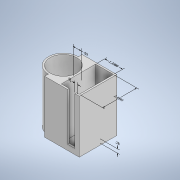
# Autodesk Inventor part: piCaseHolderForMeade
Saved by Autodesk Inventor 2021.2 (Build 252289000, 289)
## iProperties
Created: 2021-02-07
Part Number: piCaseHolderForMeade
Material: Generic
Document SubType Name: Modeling
Designer: robst
Density: 1 g/cm^3
Appearance: Default
Author: robst
Autodesk Inventor part; units mm, degrees
ref_plane "XZ Plane" through (0, 0, 0) normal (0, 1, 0) x (-1, 0, 0)
ref_plane "XY Plane" through (0, 0, 0) normal (0, 0, 1) x (1, 0, 0)
sketch "Sketch1" plane through (0, 0, 0) normal (0, 1, 0) x (-1, 0, 0)
  circle A0 centre (0, 0) radius 25.4
  circle A1 centre (0, 0) radius 28.575
  dimension "d0" = 50.8
  dimension "d1" = 3.175
  constraints: 2 centre point, 2 coincident
  measures "d0" diameter of A0
  measures "d1" radial gap between concentric circles of A0 A1
extrude "Extrusion1" add sketch "Sketch1" against normal blind 100.35
ref_plane "Work Plane1" through (28.575, 0, 0) normal (1, 0, 0) x (0, 1, 0)
sketch "Sketch5" plane through (28.575, 0, 0) normal (1, 0, 0) x (0, 1, 0)
  line L0 (0, 0) -> (-100.35, 0) construction
  line L1 (-100.35, 28.575) -> (-100.35, -28.575) construction
  line L2 (0, -28.575) -> (0, 28.575) projected
  line L3 (-3.175, 0) -> (-3.175, -32.5)
  line L4 (-3.175, -32.5) -> (-97.175, -32.5)
  line L5 (-97.175, -32.5) -> (-97.175, 0)
  line L6 (-3.175, 0) -> (-3.175, 32.5)
  line L7 (-3.175, 32.5) -> (-97.175, 32.5)
  line L8 (-97.175, 32.5) -> (-97.175, 0)
  line L9 (-97.175, 32.5) -> (-3.175, -32.5) construction
  line L10 (-97.175, -32.5) -> (-3.175, 32.5) construction
  line L11 (-100.35, 35.675) -> (-100.35, -35.675)
  line L12 (-100.35, -35.675) -> (0, -35.675)
  line L13 (0, -35.675) -> (0, 35.675)
  line L14 (0, 35.675) -> (-100.35, 35.675)
  line L15 (-100.35, 35.675) -> (0, -35.675) construction
  line L16 (-100.35, -35.675) -> (0, 35.675) construction
  point P0 (-50.175, 0)
  dimension "d7" = 3.175
  dimension "d8" = 32.5
  dimension "d9" = 94
  dimension "d10" = 3.175
  dimension "d11" = 3.175
  constraints: 30 end point, 4 midpoint, 3 parallel, 3 perpendicular, 2 symmetric about line, 2 vertical, 1 point on line
  measures "d7" distance between parallel lines of L3 L2
  measures "d8" distance from line of L3.end L0
  measures "d9" distance of L3.end L4.end
  measures "d10" distance between parallel lines of L13 L6
  measures "d11" distance between parallel lines of L14 L7
extrude "Extrusion2" add sketch "Sketch5" along normal blind 34
sketch "Sketch6" plane through (0, 0, 0) normal (0, 1, 0) x (-1, 0, 0)
  circle A0 centre (0, 0) radius 28.575 projected
  line L0 (-28.575, -35.675) -> (-28.575, 0) projected
  circle A1 centre (0, 0) radius 28.575 projected
  line L1 (-28.575, 0) -> (-28.575, 48.654)
  line L2 (-28.575, 35.675) -> (-62.575, 35.675) projected
  line L3 (-28.575, 48.654) -> (-28.575, 35.675)
  line L4 (-28.575, 35.675) -> (-28.575, 0)
  line L5 (-28.575, 0) -> (-28.575, -35.675)
  line L6 (-28.575, -35.675) -> (-62.575, -35.675) projected
  line L7 (-28.575, -35.675) -> (-28.575, 35.675)
  line L8 (-28.575, 35.675) -> (0, 28.575)
  line L9 (-28.575, 35.675) -> (-28.575, -35.675) projected
  line L10 (-28.575, -35.675) -> (0, -28.575)
  arc A2 (0, 28.575) -> (0, -28.575) centre (0, 0) ccw
  point P0 (0, 28.575)
  point P1 (-28.575, 0)
  point P2 (0, -28.575)
  constraints: 14 end point, 5 point on circle, 3 collinear, 3 vertical, 1 centre point, 1 coincident, 1 concentric, 1 other
extrude "Extrusion3" add sketch "Sketch6" against normal blind 100.35 contours A0 L1 L8 | L10 L0 A0
sketch "Sketch8" plane through (62.575, 0, 0) normal (1, 0, 0) x (0, 0, -1)
  line L0 (-35.675, 0) -> (-35.675, -100.35) projected
  line L1 (35.675, -100.35) -> (35.675, 0) projected
  line L2 (-35.675, -100.35) -> (35.675, -100.35)
  line L3 (35.675, -100.35) -> (35.675, 0)
  line L4 (35.675, 0) -> (-35.675, 0)
  line L5 (-35.675, 0) -> (-35.675, -100.35)
  point P0 (0, 0)
  point P1 (35.675, -100.35)
  point P2 (-35.675, 0)
  constraints: 8 end point, 2 parallel, 1 horizontal, 1 perpendicular
extrude "Extrusion4" add sketch "Sketch8" along normal blind 3.175
sketch "Sketch9" plane through (0, 0, 0) normal (0, 1, 0) x (1, 0, 0)
  line L0 (62.575, -32.5) -> (62.575, 32.5) projected
  line L1 (28.575, 32.5) -> (62.575, 32.5) projected
  line L2 (28.575, -32.5) -> (28.575, 32.5) projected
  line L3 (28.575, -32.5) -> (62.575, -32.5) projected
  line L4 (28.575, 32.5) -> (28.575, -32.5) projected
  line L5 (28.575, -32.5) -> (62.575, -32.5)
  line L6 (62.575, -32.5) -> (62.575, 32.5)
  line L7 (62.575, 32.5) -> (28.575, 32.5)
  line L8 (28.575, 32.5) -> (28.575, -32.5)
  point P0 (0, 0)
  point P1 (28.575, 0)
  constraints: 8 end point, 2 parallel, 1 horizontal, 1 perpendicular
extrude "Extrusion5" cut sketch "Sketch9" against normal blind 3.175
sketch "Sketch10" plane through (28.575, -100.35, 35.675) normal (0, 0, 1) x (1, 0, 0)
  line L0 (0, 100.35) -> (34, 100.35) projected
  line L1 (15, 100.35) -> (15, 10.35)
  line L2 (15, 10.35) -> (29, 10.35)
  line L3 (29, 10.35) -> (29, 100.35)
  line L4 (15, 100.35) -> (29, 100.35)
  line L5 (34, 3.175) -> (34, 100.35) projected
  line L6 (0, 100.35) -> (0, 0) projected
  point P0 (-28.575, 100.35)
  dimension "d29" = 15
  dimension "d30" = 5
  dimension "d31" = 90
  constraints: 8 end point, 3 perpendicular, 2 point on line, 1 vertical
  measures "d29" distance between parallel lines of L1 L6
  measures "d30" distance between parallel lines of L3 L5
  measures "d31" distance between parallel lines of L2 L0
extrude "Extrusion6" cut sketch "Sketch10" against normal up to surface (3.175 mm away)
sketch "Sketch11" plane through (0, 0, 0) normal (0, 1, 0) x (1, 0, 0)
  arc A0 (28.575, 0) -> (0, 28.575) centre (0, 0) ccw projected
  line L0 (0, 28.575) -> (0, 35.675)
  line L1 (28.575, 35.675) -> (0, 28.575) projected
  line L2 (0, 35.675) -> (28.575, 35.675)
  line L3 (0, -28.575) -> (28.575, -35.675) projected
  line L4 (28.575, -35.675) -> (0, -28.575) projected
  line L5 (0, -28.575) -> (0, -35.675)
  line L6 (0, -35.675) -> (28.575, -35.675)
  line L7 (28.575, -35.675) -> (0, -28.575)
  constraints: 10 end point, 2 horizontal, 2 vertical, 1 collinear
extrude "Extrusion8" add sketch "Sketch11" against normal blind 100.35
equation "\"d0\" = legDiameter"
equation "\"d1\" = legPartThickness"
equation "\"d2\" = piBoxExteriorLength"
equation "\"d7\" = piBoxWallThickness"
equation "\"d8\" = 0.5 * piBoxInteriorWidth"
equation "\"d9\" = piBoxInteriorLength"
equation "\"d10\" = piBoxWallThickness"
equation "\"d11\" = piBoxWallThickness"
equation "\"d12\" = piBoxInteriorHeight"
equation "\"d14\" = piBoxExteriorLength"
equation "\"d19\" = piBoxThickness"
equation "\"d21\" = piBoxWallThickness"
equation "\"d44\" = piBoxExteriorLength"
equation "\"legDiameter\" = 50.8"
equation "\"legPartThickness\" = 3.175"
equation "\"legPartHeight\" = piBoxExteriorLength"
equation "\"piBoxInteriorLength\" = 94"
equation "\"piBoxInteriorWidth\" = 65"
equation "\"piBoxInteriorHeight\" = 34"
equation "\"piBoxThickness\" = 3.175"
equation "\"piBoxWallThickness\" = 3.175"
equation "\"piBoxExteriorLength\" = piBoxInteriorLength + 2 * piBoxWallThickness"
equation "\"piBoxExteriorHeight\" = piBoxInteriorHeight + piBoxWallThickness"
body "Solid1"
